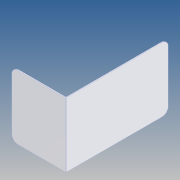
# Autodesk Inventor part: book_stand
Saved by Autodesk Inventor 2020 (Build 240168000, 168)
## iProperties
Created: 2021-04-15
Part Number: book_stand
Material: Generic
Document SubType Name: Modeling
Designer: stephen
Density: 1 g/cm^3
Appearance: PTFE
Author: stephen
Autodesk Inventor part; units mm, degrees
ref_plane "YZ Plane" through (0, 0, 0) normal (1, 0, 0) x (0, 1, 0)
ref_plane "XZ Plane" through (0, 0, 0) normal (0, 1, 0) x (-1, 0, 0)
ref_plane "XY Plane" through (0, 0, 0) normal (0, 0, 1) x (1, 0, 0)
sketch "Sketch1" plane through (0, 0, 0) normal (0, 1, 0) x (-1, 0, 0)
  line L0 (0, 0) -> (0, -205.74)
  line L1 (0, 0) -> (109.22, 0)
  line L2 (1.5875, -205.74) -> (1.5875, -1.5875)
  line L3 (1.5875, -1.5875) -> (109.22, -1.5875)
  line L4 (109.22, 0) -> (109.22, -1.5875)
  line L5 (0, -205.74) -> (1.5875, -205.74)
  dimension "d0" = 205.74
  dimension "d1" = 109.22
  dimension "d2" = 1.5875
  constraints: 12 end point, 2 vertical, 1 horizontal, 1 perpendicular, 1 other
  measures "d0" distance of L0.start L0.end
  measures "d1" distance of L0.start L1.end
  measures "d2" distance between parallel lines of L1 L3
extrude "Extrusion1" add sketch "Sketch1" along normal blind 129.54
fillet "Fillet1" radius 12.7 4 edges at (-0.7938, 129.54, -205.74) (-0.7938, 0, -205.74) (-109.22, 129.54, -0.7937) (-109.22, 0, -0.7937)
fillet "Fillet2" radius 1.27 2 edges at (0, 64.77, 0) (-1.5875, 64.77, -1.5875)
body "Solid1"
